Autodesk Fusion 360 part; units mm, degrees
(part 7 of 19)
  spline S237 degree 5 poles (-22.6635, 17.8166) (-22.6656, 17.8176) (-22.6751, 17.8223) (-22.6921, 17.8306) (-22.7166, 17.8424) (-22.7487, 17.8576) (-22.7863, 17.8752) (-22.824, 17.8925) (-22.8618, 17.9096) (-22.8998, 17.9265) (-22.938, 17.9432) (-22.9762, 17.9597) (-23.0146, 17.976) (-23.0531, 17.9922) (-23.0917, 18.0081) (-23.1305, 18.0238) (-23.1694, 18.0394) (-23.2084, 18.0547) (-23.2475, 18.0699) (-23.2867, 18.0849) (-23.3261, 18.0998) (-23.3655, 18.1144) (-23.405, 18.1289) (-23.4447, 18.1432) (-23.4845, 18.1574) (-23.5243, 18.1713) (-23.5643, 18.1851) (-23.6044, 18.1988) (-23.6445, 18.2123) (-23.6848, 18.2256) (-23.7251, 18.2388) (-23.7656, 18.2518) (-23.8061, 18.2646) (-23.8467, 18.2773) (-23.8874, 18.2899) (-23.9283, 18.3022) (-23.9692, 18.3145) (-24.0101, 18.3265) (-24.0512, 18.3385) (-24.0924, 18.3503) (-24.1336, 18.3619) (-24.1749, 18.3734) (-24.2163, 18.3847) (-24.2578, 18.3959) (-24.2994, 18.407) (-24.341, 18.4179) (-24.3827, 18.4286) (-24.4245, 18.4392) (-24.4664, 18.4497) (-24.5083, 18.46) (-24.5504, 18.4702) (-24.5925, 18.4803) (-24.6347, 18.4902) (-24.6769, 18.5) (-24.7192, 18.5096) (-24.7616, 18.5191) (-24.7956, 18.5266) (-24.8211, 18.5322) (-24.8381, 18.5358) (-24.8466, 18.5377) knots 0.224488 0.224488 0.224488 0.224488 0.224488 0.224488 0.228571 0.242857 0.257143 0.271429 0.285714 0.3 0.314286 0.328571 0.342857 0.357143 0.371429 0.385714 0.4 0.414286 0.428571 0.442857 0.457143 0.471429 0.485714 0.5 0.514286 0.528571 0.542857 0.557143 0.571429 0.585714 0.6 0.614286 0.628571 0.642857 0.657143 0.671429 0.685714 0.7 0.714286 0.728571 0.742857 0.757143 0.771429 0.785714 0.8 0.814286 0.828571 0.842857 0.857143 0.871429 0.885714 0.9 0.914286 0.928571 0.942857 0.957143 0.971429 0.985714 1 1 1 1 1 1
  arc A149 (-24.8466, 18.5377) -> (-25.3084, 17.9021) centre (0, 0) ccw
  spline S238 degree 5 poles (-25.3084, 17.9021) (-25.304, 17.8946) (-25.2953, 17.8795) (-25.2821, 17.857) (-25.2645, 17.827) (-25.2424, 17.7896) (-25.2201, 17.7523) (-25.1978, 17.7152) (-25.1753, 17.6781) (-25.1527, 17.6412) (-25.13, 17.6044) (-25.1072, 17.5677) (-25.0843, 17.5311) (-25.0613, 17.4946) (-25.0382, 17.4582) (-25.015, 17.422) (-24.9916, 17.3859) (-24.9682, 17.3499) (-24.9446, 17.314) (-24.9209, 17.2783) (-24.8971, 17.2426) (-24.8732, 17.2072) (-24.8491, 17.1718) (-24.825, 17.1365) (-24.8007, 17.1014) (-24.7763, 17.0664) (-24.7518, 17.0316) (-24.7272, 16.9969) (-24.7024, 16.9623) (-24.6776, 16.9278) (-24.6526, 16.8935) (-24.6275, 16.8594) (-24.6022, 16.8253) (-24.5769, 16.7915) (-24.5514, 16.7577) (-24.5258, 16.7241) (-24.5, 16.6907) (-24.4742, 16.6574) (-24.4482, 16.6242) (-24.422, 16.5913) (-24.3958, 16.5584) (-24.3694, 16.5258) (-24.3429, 16.4933) (-24.3162, 16.4609) (-24.2894, 16.4288) (-24.2625, 16.3967) (-24.2354, 16.3649) (-24.2081, 16.3333) (-24.1808, 16.3018) (-24.1532, 16.2705) (-24.1256, 16.2394) (-24.0977, 16.2085) (-24.0698, 16.1778) (-24.0416, 16.1473) (-24.0133, 16.117) (-23.9889, 16.0912) (-23.9701, 16.0715) (-23.957, 16.0579) (-23.9496, 16.0503) (-23.948, 16.0486) knots -1 -1 -1 -1 -1 -1 -0.985714 -0.971429 -0.957143 -0.942857 -0.928571 -0.914286 -0.9 -0.885714 -0.871429 -0.857143 -0.842857 -0.828571 -0.814286 -0.8 -0.785714 -0.771429 -0.757143 -0.742857 -0.728571 -0.714286 -0.7 -0.685714 -0.671429 -0.657143 -0.642857 -0.628571 -0.614286 -0.6 -0.585714 -0.571429 -0.557143 -0.542857 -0.528571 -0.514286 -0.5 -0.485714 -0.471429 -0.457143 -0.442857 -0.428571 -0.414286 -0.4 -0.385714 -0.371429 -0.357143 -0.342857 -0.328571 -0.314286 -0.3 -0.285714 -0.271429 -0.257143 -0.242857 -0.228571 -0.224488 -0.224488 -0.224488 -0.224488 -0.224488 -0.224488
  spline S239 degree 3 poles (-23.9365, 15.9236) (-23.9293, 15.9344) (-23.9242, 15.9466) (-23.9191, 15.9721) (-23.9191, 15.9853) (-23.9234, 16.0075) (-23.9266, 16.0167) (-23.9356, 16.0338) (-23.9412, 16.0417) (-23.948, 16.0486) knots 0 0 0 0 0.003906 0.003906 0.007813 0.007813 0.010709 0.010709 0.013605 0.013605 0.013605 0.013605
  arc A150 (-23.9365, 15.9236) -> (-24.2828, 15.3904) centre (0, 0) ccw
  spline S240 degree 3 poles (-24.4016, 15.35) (-24.3894, 15.3455) (-24.3764, 15.3435) (-24.3504, 15.3445) (-24.3376, 15.3475) (-24.317, 15.3569) (-24.3088, 15.3622) (-24.2943, 15.3748) (-24.2879, 15.3822) (-24.2828, 15.3904) knots 0 0 0 0 0.003906 0.003906 0.007813 0.007813 0.010709 0.010709 0.013605 0.013605 0.013605 0.013605
  spline S241 degree 5 poles (-24.4016, 15.35) (-24.4039, 15.3508) (-24.4138, 15.3545) (-24.4316, 15.3609) (-24.4572, 15.3701) (-24.4907, 15.3819) (-24.5299, 15.3954) (-24.5692, 15.4087) (-24.6087, 15.4218) (-24.6482, 15.4346) (-24.6879, 15.4473) (-24.7276, 15.4597) (-24.7675, 15.4719) (-24.8075, 15.4839) (-24.8476, 15.4957) (-24.8878, 15.5073) (-24.9281, 15.5187) (-24.9685, 15.5299) (-25.009, 15.5409) (-25.0495, 15.5517) (-25.0902, 15.5624) (-25.131, 15.5728) (-25.1718, 15.5831) (-25.2128, 15.5932) (-25.2538, 15.6031) (-25.2949, 15.6128) (-25.3361, 15.6224) (-25.3773, 15.6318) (-25.4187, 15.641) (-25.4601, 15.65) (-25.5016, 15.6589) (-25.5432, 15.6676) (-25.5849, 15.6762) (-25.6266, 15.6845) (-25.6684, 15.6927) (-25.7103, 15.7008) (-25.7522, 15.7087) (-25.7942, 15.7164) (-25.8363, 15.724) (-25.8785, 15.7314) (-25.9207, 15.7387) (-25.963, 15.7458) (-26.0054, 15.7527) (-26.0478, 15.7595) (-26.0903, 15.7661) (-26.1329, 15.7726) (-26.1755, 15.779) (-26.2181, 15.7852) (-26.2609, 15.7912) (-26.3037, 15.7971) (-26.3466, 15.8028) (-26.3895, 15.8084) (-26.4325, 15.8139) (-26.4755, 15.8192) (-26.5186, 15.8244) (-26.5617, 15.8294) (-26.5963, 15.8333) (-26.6223, 15.8361) (-26.6396, 15.838) (-26.6482, 15.8389) knots 0.224488 0.224488 0.224488 0.224488 0.224488 0.224488 0.228571 0.242857 0.257143 0.271429 0.285714 0.3 0.314286 0.328571 0.342857 0.357143 0.371429 0.385714 0.4 0.414286 0.428571 0.442857 0.457143 0.471429 0.485714 0.5 0.514286 0.528571 0.542857 0.557143 0.571429 0.585714 0.6 0.614286 0.628571 0.642857 0.657143 0.671429 0.685714 0.7 0.714286 0.728571 0.742857 0.757143 0.771429 0.785714 0.8 0.814286 0.828571 0.842857 0.857143 0.871429 0.885714 0.9 0.914286 0.928571 0.942857 0.957143 0.971429 0.985714 1 1 1 1 1 1
  arc A151 (-26.6482, 15.8389) -> (-27.041, 15.1586) centre (0, 0) ccw
  spline S242 degree 5 poles (-27.041, 15.1586) (-27.0359, 15.1515) (-27.0256, 15.1375) (-27.0102, 15.1164) (-26.9895, 15.0884) (-26.9636, 15.0536) (-26.9376, 15.0188) (-26.9115, 14.9842) (-26.8852, 14.9497) (-26.8589, 14.9154) (-26.8325, 14.8811) (-26.806, 14.847) (-26.7794, 14.813) (-26.7527, 14.7791) (-26.7259, 14.7454) (-26.699, 14.7118) (-26.672, 14.6783) (-26.6449, 14.645) (-26.6177, 14.6118) (-26.5904, 14.5787) (-26.563, 14.5457) (-26.5355, 14.5129) (-26.5079, 14.4803) (-26.4802, 14.4477) (-26.4524, 14.4154) (-26.4245, 14.3831) (-26.3965, 14.351) (-26.3684, 14.3191) (-26.3401, 14.2873) (-26.3118, 14.2556) (-26.2834, 14.2241) (-26.2548, 14.1927) (-26.2262, 14.1615) (-26.1974, 14.1305) (-26.1685, 14.0996) (-26.1396, 14.0689) (-26.1105, 14.0383) (-26.0813, 14.0079) (-26.0519, 13.9776) (-26.0225, 13.9476) (-25.993, 13.9177) (-25.9633, 13.8879) (-25.9335, 13.8584) (-25.9036, 13.829) (-25.8736, 13.7998) (-25.8435, 13.7708) (-25.8132, 13.742) (-25.7828, 13.7134) (-25.7523, 13.6849) (-25.7217, 13.6567) (-25.6909, 13.6287) (-25.66, 13.6008) (-25.6289, 13.5732) (-25.5978, 13.5458) (-25.5665, 13.5186) (-25.5395, 13.4955) (-25.5187, 13.4779) (-25.5043, 13.4658) (-25.4961, 13.459) (-25.4943, 13.4574) knots -1 -1 -1 -1 -1 -1 -0.985714 -0.971429 -0.957143 -0.942857 -0.928571 -0.914286 -0.9 -0.885714 -0.871429 -0.857143 -0.842857 -0.828571 -0.814286 -0.8 -0.785714 -0.771429 -0.757143 -0.742857 -0.728571 -0.714286 -0.7 -0.685714 -0.671429 -0.657143 -0.642857 -0.628571 -0.614286 -0.6 -0.585714 -0.571429 -0.557143 -0.542857 -0.528571 -0.514286 -0.5 -0.485714 -0.471429 -0.457143 -0.442857 -0.428571 -0.414286 -0.4 -0.385714 -0.371429 -0.357143 -0.342857 -0.328571 -0.314286 -0.3 -0.285714 -0.271429 -0.257143 -0.242857 -0.228571 -0.224488 -0.224488 -0.224488 -0.224488 -0.224488 -0.224488
  spline S243 degree 3 poles (-25.4698, 13.3343) (-25.4638, 13.3459) (-25.4601, 13.3585) (-25.4576, 13.3844) (-25.459, 13.3975) (-25.4656, 13.4192) (-25.4698, 13.4279) (-25.4804, 13.444) (-25.4869, 13.4513) (-25.4943, 13.4574) knots 0 0 0 0 0.003906 0.003906 0.007813 0.007813 0.010709 0.010709 0.013605 0.013605 0.013605 0.013605
  arc A152 (-25.4698, 13.3343) -> (-25.7585, 12.7678) centre (0, 0) ccw
  spline S244 degree 3 poles (-25.8725, 12.7152) (-25.8598, 12.7121) (-25.8467, 12.7114) (-25.8209, 12.7151) (-25.8085, 12.7194) (-25.789, 12.731) (-25.7814, 12.737) (-25.7683, 12.7512) (-25.7628, 12.7592) (-25.7585, 12.7678) knots 0 0 0 0 0.003906 0.003906 0.007813 0.007813 0.010709 0.010709 0.013605 0.013605 0.013605 0.013605
  spline S245 degree 5 poles (-25.8725, 12.7152) (-25.8748, 12.7158) (-25.8851, 12.7184) (-25.9034, 12.723) (-25.9299, 12.7294) (-25.9644, 12.7377) (-26.0048, 12.747) (-26.0453, 12.7561) (-26.0859, 12.765) (-26.1265, 12.7736) (-26.1673, 12.7821) (-26.2082, 12.7902) (-26.2491, 12.7982) (-26.2901, 12.806) (-26.3312, 12.8135) (-26.3724, 12.8209) (-26.4137, 12.828) (-26.455, 12.8349) (-26.4964, 12.8416) (-26.5379, 12.8482) (-26.5795, 12.8545) (-26.6211, 12.8606) (-26.6628, 12.8666) (-26.7046, 12.8723) (-26.7464, 12.8779) (-26.7883, 12.8833) (-26.8303, 12.8885) (-26.8723, 12.8935) (-26.9144, 12.8983) (-26.9565, 12.903) (-26.9987, 12.9075) (-27.041, 12.9118) (-27.0833, 12.9159) (-27.1257, 12.9199) (-27.1681, 12.9237) (-27.2106, 12.9273) (-27.2532, 12.9308) (-27.2958, 12.9341) (-27.3384, 12.9372) (-27.3811, 12.9402) (-27.4239, 12.943) (-27.4667, 12.9456) (-27.5095, 12.9481) (-27.5524, 12.9504) (-27.5954, 12.9526) (-27.6384, 12.9546) (-27.6814, 12.9565) (-27.7245, 12.9581) (-27.7677, 12.9597) (-27.8108, 12.9611) (-27.8541, 12.9623) (-27.8973, 12.9634) (-27.9407, 12.9643) (-27.984, 12.9651) (-28.0274, 12.9657) (-28.0708, 12.9662) (-28.1056, 12.9665) (-28.1317, 12.9666) (-28.1492, 12.9667) (-28.1579, 12.9667) knots 0.224488 0.224488 0.224488 0.224488 0.224488 0.224488 0.228571 0.242857 0.257143 0.271429 0.285714 0.3 0.314286 0.328571 0.342857 0.357143 0.371429 0.385714 0.4 0.414286 0.428571 0.442857 0.457143 0.471429 0.485714 0.5 0.514286 0.528571 0.542857 0.557143 0.571429 0.585714 0.6 0.614286 0.628571 0.642857 0.657143 0.671429 0.685714 0.7 0.714286 0.728571 0.742857 0.757143 0.771429 0.785714 0.8 0.814286 0.828571 0.842857 0.857143 0.871429 0.885714 0.9 0.914286 0.928571 0.942857 0.957143 0.971429 0.985714 1 1 1 1 1 1
  arc A153 (-28.1579, 12.9667) -> (-28.4774, 12.249) centre (0, 0) ccw
  spline S246 degree 5 poles (-28.4774, 12.249) (-28.4716, 12.2425) (-28.4599, 12.2296) (-28.4423, 12.2103) (-28.4188, 12.1846) (-28.3894, 12.1527) (-28.3599, 12.1208) (-28.3303, 12.0891) (-28.3006, 12.0576) (-28.2709, 12.0261) (-28.241, 11.9948) (-28.2111, 11.9637) (-28.1811, 11.9326) (-28.151, 11.9018) (-28.1208, 11.871) (-28.0906, 11.8404) (-28.0602, 11.8099) (-28.0298, 11.7796) (-27.9993, 11.7494) (-27.9687, 11.7194) (-27.938, 11.6895) (-27.9072, 11.6597) (-27.8763, 11.6301) (-27.8454, 11.6007) (-27.8143, 11.5714) (-27.7832, 11.5422) (-27.752, 11.5132) (-27.7207, 11.4844) (-27.6893, 11.4557) (-27.6578, 11.4272) (-27.6262, 11.3988) (-27.5946, 11.3706) (-27.5628, 11.3426) (-27.5309, 11.3147) (-27.499, 11.287) (-27.467, 11.2595) (-27.4348, 11.2321) (-27.4026, 11.2049) (-27.3703, 11.1779) (-27.3379, 11.1511) (-27.3054, 11.1244) (-27.2728, 11.098) (-27.2401, 11.0717) (-27.2073, 11.0456) (-27.1743, 11.0197) (-27.1413, 10.994) (-27.1082, 10.9685) (-27.075, 10.9432) (-27.0417, 10.9181) (-27.0083, 10.8932) (-26.9747, 10.8686) (-26.9411, 10.8441) (-26.9073, 10.8199) (-26.8735, 10.7959) (-26.8395, 10.7721) (-26.8103, 10.752) (-26.7878, 10.7367) (-26.7721, 10.7261) (-26.7633, 10.7202) (-26.7613, 10.7188) knots -1 -1 -1 -1 -1 -1 -0.985714 -0.971429 -0.957143 -0.942857 -0.928571 -0.914286 -0.9 -0.885714 -0.871429 -0.857143 -0.842857 -0.828571 -0.814286 -0.8 -0.785714 -0.771429 -0.757143 -0.742857 -0.728571 -0.714286 -0.7 -0.685714 -0.671429 -0.657143 -0.642857 -0.628571 -0.614286 -0.6 -0.585714 -0.571429 -0.557143 -0.542857 -0.528571 -0.514286 -0.5 -0.485714 -0.471429 -0.457143 -0.442857 -0.428571 -0.414286 -0.4 -0.385714 -0.371429 -0.357143 -0.342857 -0.328571 -0.314286 -0.3 -0.285714 -0.271429 -0.257143 -0.242857 -0.228571 -0.224488 -0.224488 -0.224488 -0.224488 -0.224488 -0.224488
  spline S247 degree 3 poles (-26.7241, 10.599) (-26.7193, 10.6111) (-26.7169, 10.624) (-26.7172, 10.65) (-26.7199, 10.6629) (-26.7288, 10.6838) (-26.7338, 10.6921) (-26.7461, 10.7069) (-26.7533, 10.7135) (-26.7613, 10.7188) knots 0 0 0 0 0.003906 0.003906 0.007813 0.007813 0.010709 0.010709 0.013605 0.013605 0.013605 0.013605
  arc A154 (-26.7241, 10.599) -> (-26.952, 10.0054) centre (0, 0) ccw
  spline S248 degree 3 poles (-27.0598, 9.9412) (-27.047, 9.9393) (-27.0338, 9.94) (-27.0086, 9.9464) (-26.9967, 9.952) (-26.9785, 9.9655) (-26.9716, 9.9724) (-26.96, 9.9878) (-26.9553, 9.9963) (-26.952, 10.0054) knots 0 0 0 0 0.003906 0.003906 0.007813 0.007813 0.010709 0.010709 0.013605 0.013605 0.013605 0.013605
  spline S249 degree 5 poles (-27.0598, 9.9412) (-27.0622, 9.9415) (-27.0727, 9.943) (-27.0914, 9.9456) (-27.1184, 9.9493) (-27.1536, 9.9539) (-27.1948, 9.9589) (-27.236, 9.9638) (-27.2773, 9.9683) (-27.3186, 9.9727) (-27.3601, 9.9768) (-27.4015, 9.9807) (-27.4431, 9.9843) (-27.4847, 9.9878) (-27.5264, 9.991) (-27.5681, 9.994) (-27.6099, 9.9967) (-27.6517, 9.9993) (-27.6936, 10.0016) (-27.7355, 10.0038) (-27.7775, 10.0057) (-27.8196, 10.0075) (-27.8617, 10.0091) (-27.9038, 10.0104) (-27.946, 10.0116) (-27.9882, 10.0126) (-28.0305, 10.0133) (-28.0728, 10.0139) (-28.1152, 10.0144) (-28.1576, 10.0146) (-28.2, 10.0146) (-28.2425, 10.0145) (-28.285, 10.0142) (-28.3276, 10.0137) (-28.3702, 10.0131) (-28.4128, 10.0122) (-28.4555, 10.0112) (-28.4982, 10.01) (-28.541, 10.0087) (-28.5837, 10.0072) (-28.6265, 10.0055) (-28.6694, 10.0037) (-28.7123, 10.0016) (-28.7552, 9.9995) (-28.7981, 9.9971) (-28.8411, 9.9946) (-28.8841, 9.992) (-28.9271, 9.9892) (-28.9702, 9.9862) (-29.0133, 9.983) (-29.0564, 9.9798) (-29.0996, 9.9763) (-29.1427, 9.9727) (-29.1859, 9.9689) (-29.2292, 9.965) (-29.2724, 9.961) (-29.307, 9.9576) (-29.333, 9.955) (-29.3503, 9.9532) (-29.359, 9.9524) knots 0.224488 0.224488 0.224488 0.224488 0.224488 0.224488 0.228571 0.242857 0.257143 0.271429 0.285714 0.3 0.314286 0.328571 0.342857 0.357143 0.371429 0.385714 0.4 0.414286 0.428571 0.442857 0.457143 0.471429 0.485714 0.5 0.514286 0.528571 0.542857 0.557143 0.571429 0.585714 0.6 0.614286 0.628571 0.642857 0.657143 0.671429 0.685714 0.7 0.714286 0.728571 0.742857 0.757143 0.771429 0.785714 0.8 0.814286 0.828571 0.842857 0.857143 0.871429 0.885714 0.9 0.914286 0.928571 0.942857 0.957143 0.971429 0.985714 1 1 1 1 1 1
  arc A155 (-29.359, 9.9524) -> (-29.6018, 9.2052) centre (0, 0) ccw
  spline S250 degree 5 poles (-29.6018, 9.2052) (-29.5953, 9.1994) (-29.5823, 9.1877) (-29.5628, 9.1704) (-29.5368, 9.1473) (-29.5042, 9.1186) (-29.4715, 9.09) (-29.4388, 9.0616) (-29.406, 9.0333) (-29.3731, 9.0051) (-29.3401, 8.9771) (-29.3071, 8.9493) (-29.274, 8.9215) (-29.2409, 8.894) (-29.2076, 8.8665) (-29.1743, 8.8393) (-29.141, 8.8121) (-29.1075, 8.7851) (-29.074, 8.7583) (-29.0405, 8.7316) (-29.0068, 8.7051) (-28.9731, 8.6787) (-28.9393, 8.6525) (-28.9054, 8.6265) (-28.8715, 8.6006) (-28.8375, 8.5748) (-28.8034, 8.5493) (-28.7693, 8.5239) (-28.735, 8.4986) (-28.7007, 8.4735) (-28.6664, 8.4486) (-28.6319, 8.4239) (-28.5974, 8.3993) (-28.5628, 8.3749) (-28.5282, 8.3507) (-28.4934, 8.3267) (-28.4586, 8.3028) (-28.4237, 8.2792) (-28.3888, 8.2557) (-28.3537, 8.2324) (-28.3186, 8.2093) (-28.2834, 8.1864) (-28.2481, 8.1637) (-28.2128, 8.1412) (-28.1774, 8.1188) (-28.1418, 8.0967) (-28.1062, 8.0748) (-28.0706, 8.0531) (-28.0348, 8.0317) (-27.999, 8.0104) (-27.963, 7.9894) (-27.927, 7.9686) (-27.8909, 7.9481) (-27.8547, 7.9277) (-27.8185, 7.9076) (-27.7873, 7.8907) (-27.7633, 7.8778) (-27.7466, 7.8689) (-27.7372, 7.8639) (-27.7352, 7.8628) knots -1 -1 -1 -1 -1 -1 -0.985714 -0.971429 -0.957143 -0.942857 -0.928571 -0.914286 -0.9 -0.885714 -0.871429 -0.857143 -0.842857 -0.828571 -0.814286 -0.8 -0.785714 -0.771429 -0.757143 -0.742857 -0.728571 -0.714286 -0.7 -0.685714 -0.671429 -0.657143 -0.642857 -0.628571 -0.614286 -0.6 -0.585714 -0.571429 -0.557143 -0.542857 -0.528571 -0.514286 -0.5 -0.485714 -0.471429 -0.457143 -0.442857 -0.428571 -0.414286 -0.4 -0.385714 -0.371429 -0.357143 -0.342857 -0.328571 -0.314286 -0.3 -0.285714 -0.271429 -0.257143 -0.242857 -0.228571 -0.224488 -0.224488 -0.224488 -0.224488 -0.224488 -0.224488
  spline S251 degree 3 poles (-27.6856, 7.7475) (-27.6821, 7.76) (-27.6811, 7.7731) (-27.6841, 7.799) (-27.6881, 7.8115) (-27.6991, 7.8313) (-27.705, 7.839) (-27.7188, 7.8526) (-27.7266, 7.8583) (-27.7352, 7.8628) knots 0 0 0 0 0.003906 0.003906 0.007813 0.007813 0.010709 0.010709 0.013605 0.013605 0.013605 0.013605
  arc A156 (-27.6856, 7.7475) -> (-27.8502, 7.1333) centre (0, 0) ccw
  spline S252 degree 3 poles (-27.9507, 7.0582) (-27.9377, 7.0577) (-27.9248, 7.0598) (-27.9003, 7.0688) (-27.8891, 7.0756) (-27.8724, 7.0909) (-27.8662, 7.0984) (-27.8563, 7.115) (-27.8526, 7.124) (-27.8502, 7.1333) knots 0 0 0 0 0.003906 0.003906 0.007813 0.007813 0.010709 0.010709 0.013605 0.013605 0.013605 0.013605
  spline S253 degree 5 poles (-27.9507, 7.0582) (-27.9531, 7.0583) (-27.9637, 7.0587) (-27.9826, 7.0593) (-28.0098, 7.0601) (-28.0453, 7.061) (-28.0868, 7.0618) (-28.1283, 7.0622) (-28.1698, 7.0625) (-28.2114, 7.0625) (-28.253, 7.0622) (-28.2947, 7.0618) (-28.3364, 7.0611) (-28.3781, 7.0601) (-28.4199, 7.059) (-28.4617, 7.0576) (-28.5036, 7.0559) (-28.5454, 7.0541) (-28.5873, 7.0521) (-28.6293, 7.0498) (-28.6712, 7.0474) (-28.7132, 7.0447) (-28.7553, 7.0419) (-28.7973, 7.0388) (-28.8394, 7.0356) (-28.8815, 7.0321) (-28.9236, 7.0285) (-28.9658, 7.0247) (-29.0079, 7.0207) (-29.0501, 7.0165) (-29.0923, 7.0121) (-29.1346, 7.0075) (-29.1768, 7.0027) (-29.2191, 6.9978) (-29.2614, 6.9927) (-29.3037, 6.9874) (-29.3461, 6.982) (-29.3884, 6.9763) (-29.4308, 6.9705) (-29.4732, 6.9646) (-29.5156, 6.9584) (-29.558, 6.9521) (-29.6004, 6.9456) (-29.6429, 6.939) (-29.6854, 6.9321) (-29.7278, 6.9252) (-29.7703, 6.918) (-29.8128, 6.9107) (-29.8553, 6.9033) (-29.8979, 6.8956) (-29.9404, 6.8879) (-29.983, 6.8799) (-30.0255, 6.8718) (-30.0681, 6.8636) (-30.1107, 6.8552) (-30.1533, 6.8466) (-30.1873, 6.8396) (-30.2129, 6.8343) (-30.2299, 6.8308) (-30.2385, 6.829) knots 0.224488 0.224488 0.224488 0.224488 0.224488 0.224488 0.228571 0.242857 0.257143 0.271429 0.285714 0.3 0.314286 0.328571 0.342857 0.357143 0.371429 0.385714 0.4 0.414286 0.428571 0.442857 0.457143 0.471429 0.485714 0.5 0.514286 0.528571 0.542857 0.557143 0.571429 0.585714 0.6 0.614286 0.628571 0.642857 0.657143 0.671429 0.685714 0.7 0.714286 0.728571 0.742857 0.757143 0.771429 0.785714 0.8 0.814286 0.828571 0.842857 0.857143 0.871429 0.885714 0.9 0.914286 0.928571 0.942857 0.957143 0.971429 0.985714 1 1 1 1 1 1
  arc A157 (-30.2385, 6.829) -> (-30.4018, 6.0605) centre (0, 0) ccw
  spline S254 degree 5 poles (-30.4018, 6.0605) (-30.3948, 6.0554) (-30.3806, 6.0452) (-30.3594, 6.03) (-30.3311, 6.0097) (-30.2957, 5.9846) (-30.2602, 5.9596) (-30.2247, 5.9348) (-30.1891, 5.91) (-30.1535, 5.8855) (-30.1178, 5.8611) (-30.082, 5.8368) (-30.0462, 5.8127) (-30.0104, 5.7887) (-29.9744, 5.7649) (-29.9385, 5.7413) (-29.9025, 5.7178) (-29.8664, 5.6945) (-29.8303, 5.6713) (-29.7941, 5.6483) (-29.7578, 5.6254) (-29.7215, 5.6027) (-29.6852, 5.5802) (-29.6488, 5.5578) (-29.6123, 5.5356) (-29.5758, 5.5135) (-29.5393, 5.4917) (-29.5026, 5.47) (-29.466, 5.4484) (-29.4292, 5.4271) (-29.3925, 5.4059) (-29.3556, 5.3849) (-29.3187, 5.3641) (-29.2818, 5.3434) (-29.2448, 5.323) (-29.2077, 5.3027) (-29.1706, 5.2826) (-29.1334, 5.2627) (-29.0962, 5.243) (-29.0589, 5.2235) (-29.0216, 5.2042) (-28.9842, 5.1851) (-28.9467, 5.1662) (-28.9092, 5.1475) (-28.8716, 5.129) (-28.834, 5.1107) (-28.7963, 5.0927) (-28.7586, 5.0749) (-28.7208, 5.0572) (-28.6829, 5.0399) (-28.645, 5.0227) (-28.607, 5.0058) (-28.5689, 4.9891) (-28.5308, 4.9727) (-28.4926, 4.9565) (-28.4599, 4.9429) (-28.4347, 4.9326) (-28.4172, 4.9255) (-28.4073, 4.9215) (-28.4051, 4.9206) knots -1 -1 -1 -1 -1 -1 -0.985714 -0.971429 -0.957143 -0.942857 -0.928571 -0.914286 -0.9 -0.885714 -0.871429 -0.857143 -0.842857 -0.828571 -0.814286 -0.8 -0.785714 -0.771429 -0.757143 -0.742857 -0.728571 -0.714286 -0.7 -0.685714 -0.671429 -0.657143 -0.642857 -0.628571 -0.614286 -0.6 -0.585714 -0.571429 -0.557143 -0.542857 -0.528571 -0.514286 -0.5 -0.485714 -0.471429 -0.457143 -0.442857 -0.428571 -0.414286 -0.4 -0.385714 -0.371429 -0.357143 -0.342857 -0.328571 -0.314286 -0.3 -0.285714 -0.271429 -0.257143 -0.242857 -0.228571 -0.224488 -0.224488 -0.224488 -0.224488 -0.224488 -0.224488
  spline S255 degree 3 poles (-28.3438, 4.8111) (-28.3416, 4.8239) (-28.342, 4.8371) (-28.3477, 4.8625) (-28.353, 4.8745) (-28.366, 4.8931) (-28.3726, 4.9001) (-28.3878, 4.9121) (-28.3961, 4.917) (-28.4051, 4.9206) knots 0 0 0 0 0.003906 0.003906 0.007813 0.007813 0.010709 0.010709 0.013605 0.013605 0.013605 0.013605
  arc A158 (-28.3438, 4.8111) -> (-28.4432, 4.1831) centre (0, 0) ccw
  spline S256 degree 3 poles (-28.5354, 4.0979) (-28.5224, 4.0988) (-28.5097, 4.1022) (-28.4864, 4.1137) (-28.4759, 4.1216) (-28.4609, 4.1386) (-28.4556, 4.1467) (-28.4474, 4.1642) (-28.4447, 4.1735) (-28.4432, 4.1831) knots 0 0 0 0 0.003906 0.003906 0.007813 0.007813 0.010709 0.010709 0.013605 0.013605 0.013605 0.013605
  spline S257 degree 5 poles (-28.5354, 4.0979) (-28.5378, 4.0977) (-28.5484, 4.097) (-28.5672, 4.0957) (-28.5944, 4.0936) (-28.6298, 4.0908) (-28.6711, 4.0872) (-28.7124, 4.0833) (-28.7537, 4.0792) (-28.7951, 4.0749) (-28.8365, 4.0703) (-28.8778, 4.0655) (-28.9192, 4.0604) (-28.9607, 4.0551) (-29.0021, 4.0496) (-29.0435, 4.0438) (-29.085, 4.0379) (-29.1264, 4.0317) (-29.1679, 4.0253) (-29.2094, 4.0186) (-29.2508, 4.0118) (-29.2923, 4.0048) (-29.3338, 3.9976) (-29.3753, 3.9901) (-29.4168, 3.9825) (-29.4583, 3.9747) (-29.4998, 3.9667) (-29.5414, 3.9584) (-29.5829, 3.95) (-29.6244, 3.9415) (-29.6659, 3.9327) (-29.7075, 3.9237) (-29.749, 3.9146) (-29.7905, 3.9053) (-29.8321, 3.8958) (-29.8736, 3.8861) (-29.9151, 3.8762) (-29.9567, 3.8662) (-29.9982, 3.856) (-30.0397, 3.8456) (-30.0812, 3.8351) (-30.1228, 3.8244) (-30.1643, 3.8135) (-30.2058, 3.8024) (-30.2473, 3.7912) (-30.2889, 3.7798) (-30.3304, 3.7683) (-30.3719, 3.7566) (-30.4134, 3.7447) (-30.4549, 3.7327) (-30.4964, 3.7205) (-30.5379, 3.7082) (-30.5793, 3.6957) (-30.6208, 3.683) (-30.6623, 3.6702) (-30.7037, 3.6572) (-30.7369, 3.6467) (-30.7618, 3.6388) (-30.7784, 3.6335) (-30.7866, 3.6308) knots 0.224488 0.224488 0.224488 0.224488 0.224488 0.224488 0.228571 0.242857 0.257143 0.271429 0.285714 0.3 0.314286 0.328571 0.342857 0.357143 0.371429 0.385714 0.4 0.414286 0.428571 0.442857 0.457143 0.471429 0.485714 0.5 0.514286 0.528571 0.542857 0.557143 0.571429 0.585714 0.6 0.614286 0.628571 0.642857 0.657143 0.671429 0.685714 0.7 0.714286 0.728571 0.742857 0.757143 0.771429 0.785714 0.8 0.814286 0.828571 0.842857 0.857143 0.871429 0.885714 0.9 0.914286 0.928571 0.942857 0.957143 0.971429 0.985714 1 1 1 1 1 1
  arc A159 (-30.7866, 3.6308) -> (-30.8688, 2.8495) centre (0, 0) ccw
  spline S258 degree 5 poles (-30.8688, 2.8495) (-30.8612, 2.8451) (-30.8461, 2.8365) (-30.8234, 2.8235) (-30.7932, 2.8064) (-30.7553, 2.7851) (-30.7174, 2.7639) (-30.6795, 2.7429) (-30.6415, 2.722) (-30.6035, 2.7013) (-30.5654, 2.6808) (-30.5273, 2.6604) (-30.4892, 2.6402) (-30.451, 2.6201) (-30.4128, 2.6002) (-30.3746, 2.5804) (-30.3363, 2.5608) (-30.298, 2.5414) (-30.2596, 2.5221) (-30.2213, 2.503) (-30.1828, 2.484) (-30.1444, 2.4653) (-30.1059, 2.4466) (-30.0673, 2.4282) (-30.0287, 2.4099) (-29.9901, 2.3918) (-29.9515, 2.3739) (-29.9128, 2.3561) (-29.8741, 2.3386) (-29.8353, 2.3212) (-29.7965, 2.3039) (-29.7577, 2.2869) (-29.7188, 2.2701) (-29.6799, 2.2534) (-29.641, 2.2369) (-29.602, 2.2206) (-29.563, 2.2045) (-29.5239, 2.1886) (-29.4849, 2.1729) (-29.4457, 2.1574) (-29.4066, 2.1421) (-29.3674, 2.127) (-29.3282, 2.1122) (-29.2889, 2.0975) (-29.2496, 2.083) (-29.2103, 2.0688) (-29.1709, 2.0548) (-29.1315, 2.041) (-29.0921, 2.0274) (-29.0526, 2.0141) (-29.0131, 2.001) (-28.9735, 1.9881) (-28.9339, 1.9755) (-28.8943, 1.9632) (-28.8546, 1.9511) (-28.8206, 1.9409) (-28.7945, 1.9333) (-28.7763, 1.9281) (-28.7661, 1.9252) (-28.7638, 1.9245) knots -1 -1 -1 -1 -1 -1 -0.985714 -0.971429 -0.957143 -0.942857 -0.928571 -0.914286 -0.9 -0.885714 -0.871429 -0.857143 -0.842857 -0.828571 -0.814286 -0.8 -0.785714 -0.771429 -0.757143 -0.742857 -0.728571 -0.714286 -0.7 -0.685714 -0.671429 -0.657143 -0.642857 -0.628571 -0.614286 -0.6 -0.585714 -0.571429 -0.557143 -0.542857 -0.528571 -0.514286 -0.5 -0.485714 -0.471429 -0.457143 -0.442857 -0.428571 -0.414286 -0.4 -0.385714 -0.371429 -0.357143 -0.342857 -0.328571 -0.314286 -0.3 -0.285714 -0.271429 -0.257143 -0.242857 -0.228571 -0.224488 -0.224488 -0.224488 -0.224488 -0.224488 -0.224488
  spline S259 degree 3 poles (-28.6914, 1.822) (-28.6906, 1.835) (-28.6923, 1.848) (-28.7006, 1.8727) (-28.7072, 1.8841) (-28.7221, 1.9012) (-28.7294, 1.9075) (-28.7457, 1.9179) (-28.7546, 1.9219) (-28.7638, 1.9245) knots 0 0 0 0 0.003906 0.003906 0.007813 0.007813 0.010709 0.010709 0.013605 0.013605 0.013605 0.013605
  line L20 (0, 31) -> (0, 3.7492)
  line L21 (2.2037, 3.0332) -> (18.2213, 25.0795)
  circle A160 centre (0, 0) radius 7.5
  circle A161 centre (0, 0) radius 27.5
  dimension "d19" = 36
  dimension "d20" = 15
  dimension "d21" = 55
  constraint vertical L20
  constraint coincident A1.centre L20
  constraint coincident A1.centre L21
  constraint coincident A9 L20.end
  constraint coincident A13 L21.start
  constraint coincident A131 L20.start
  constraint coincident A119 L21.end
  constraint coincident A1.centre A3.centre
  constraint concentric A1 A161
  measures "d19" angle of L20 L21
  measures "d20" diameter of A160
  measures "d21" diameter of A161
extrude "Estrusione4" cut sketch "Schizzo1 (3)" against normal blind 1 contours L20 L21 A160 A161 picked at (8.9949, 18.7465) bodies 1 in component "Spur Gear (60 teeth)"
pattern_circular "Serie C2" count 5 over 360 about axis through (0, 0, 0) along (0, 0, 1) of "Estrusione4" in component "Spur Gear (60 teeth)"
extrude "Estrusione5" cut 1 faces at (-3.6482, -2.3787, 8) along direction (0, 0, -1) blind 1.6 on bodies 1 bodies 1 in component "Spur Gear (60 teeth)"
sketch "Schizzo2 (3)" plane through (0, 0, 2) normal (0, 0, 1) x (-1, 0, 0)
  line L0 (7.1329, -2.3176) -> (26.1541, -8.498)
  arc A0 (26.1541, -8.498) -> (26.1541, 8.498) centre (0, 0) ccw
  line L1 (26.1541, 8.498) -> (7.1329, 2.3176)
  arc A1 (7.1329, -2.3176) -> (7.1329, 2.3176) centre (0, 0) ccw
  line L2 (24.4009, 8.0452) -> (-1.5991, 8.0452) construction
  line L3 (-1.5991, 8.0452) -> (-1.5991, -2.9548) construction
  line L4 (-1.5991, -2.9548) -> (24.4009, -2.9548) construction
  line L5 (24.4009, -2.9548) -> (24.4009, 8.0452) construction
  dimension "d28" = 5
  text T0 "60s" font "Arial" height 5 bold align left top in box 26 x 11 at (24.4009, 8.0452) x (-1, 0) y (0, -1) spacing 1 kerned
extrude "Estrusione6" add sketch "Schizzo2 (3)" along normal blind 1 text T0 bodies 1 in component "Spur Gear (60 teeth)"
component "Spur Gear (60 teeth)" placed x (1, 0, 0) y (0, 1, 0) z (0, 0, 1) at (0, 0, 0)
component "Spur Gear (10 teeth)" placed x (1, 0, 0) y (0, 1, 0) z (0, 0, 1) at (0, 0, 0)
equation "d19 = ( 360 / 10 ) * 1 deg"

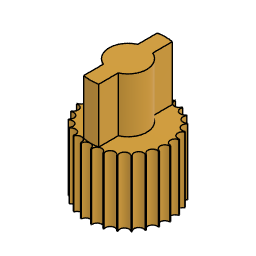
design "2 pomello lancetta secondi"
Autodesk Fusion 360 part; units mm, degrees
sketch "Schizzo1" plane through (0, 0, 0) normal (0, 0, 1) x (1, 0, 0)
  line L0 (0, -45) -> (5, 0)
  line L1 (5, 0) -> (0, 15)
  line L2 (0, 15) -> (-5, 0)
  line L3 (-5, 0) -> (0, -45)
  line L4 (0, -45) -> (0, 15) construction
  line L5 (5, 0) -> (-5, 0) construction
  line L6 (-1, 15) -> (1, 15)
  line L7 (1, 15) -> (1, -45)
  line L8 (1, -45) -> (-1, -45)
  line L9 (-1, -45) -> (-1, 15)
  circle A0 centre (0, 0) radius 5
  dimension "d1" = 45
  dimension "d2" = 15
  dimension "d3" = 5
  dimension "d12" = 1
  dimension "d13" = 1
  constraint vertical L4
  constraint perpendicular L4 L5
  constraint midpoint A0.centre L5
  constraint equal L0 L3
  constraint equal L1 L2
  constraint horizontal L6
  constraint vertical L7
  constraint horizontal L8
  constraint vertical L9
  constraint coincident A0.centre origin
  constraint coincident L0.end A0
  constraint midpoint L0.start L8
  constraint midpoint L1.end L6
  measures "d1" vertical distance of L0.start L0.end
  measures "d2" vertical distance of L0.end L1.end
  measures "d3" horizontal distance of L0.start L0.end
  measures "d12" distance of A0.centre L9
  measures "d13" distance of A0.centre L7
extrude "Estrusione1" add sketch "Schizzo1" along normal blind 2 contours L0 L3 L7 L9 A0 | L3 L8 L9 | L0 L7 L8 | L0 L1 L7 A0 | L0 A0 | L7 L9 A0 | L3 A0 | L2 L3 L9 A0 | L1 A0 | L1 L2 L7 L9 A0 | L2 A0 | L1 L6 L7 | L2 L6 L9
sketch "Schizzo2" plane through (0, 0, 2) normal (0, 0, 1) x (-1, 0, 0)
  circle A0 centre (0, 0) radius 2
  circle A1 centre (0, 0) radius 4
  line L0 (-0.8, 24) -> (0.8, 24)
  line L1 (0.8, 24) -> (0.8, -21)
  line L2 (0.8, -21) -> (-0.8, -21)
  line L3 (-0.8, -21) -> (-0.8, 24)
  arc A2 (-1, 4.899) -> (-1, -4.899) centre (0, 0) ccw
  line L4 (-1, -4.899) -> (-1, -15)
  line L5 (-1, -15) -> (1, -15)
  line L6 (1, -15) -> (1, -4.899)
  arc A3 (1, -4.899) -> (1, 4.899) centre (0, 0) ccw
  line L7 (1, 4.899) -> (1, 45)
  line L8 (-1, 45) -> (-1, 4.899)
  line L9 (1, 45) -> (-1, 45)
  dimension "d6" = 4
  dimension "d7" = 8
  dimension "d8" = 0.8
  dimension "d9" = 0.8
  constraint coincident A0.centre A1.centre
  constraint horizontal L0
  constraint vertical L1
  constraint horizontal L2
  constraint vertical L3
  measures "d6" diameter of A0
  measures "d7" diameter of A1
  measures "d8" distance of A0.centre L3
  measures "d9" distance of A0.centre L1
extrude "Estrusione2" add sketch "Schizzo2" along normal blind 3.8 contours A0 L1 | A0 L1 L3 | A0 A1 L1 L3 | A0 A1 L1 L3 | A0 L3
extrude "Estrusione3" add 1 faces at (0.3333, -45, 0.6667) along direction (0, -1, 0) blind 10
sketch "Schizzo3" plane through (0, 0, 0) normal (0, 0, -1) x (1, 0, 0)
  line L0 (1, 4.899) -> (1, 55)
  line L1 (1, 55) -> (-1, 55)
  line L2 (-1, 55) -> (-1, 4.899)
  arc A0 (-1, 4.899) -> (-1, -4.899) centre (0, 0) ccw
  line L3 (-1, -4.899) -> (-1, -15)
  line L4 (-1, -15) -> (1, -15)
  line L5 (1, -15) -> (1, -4.899)
  arc A1 (1, -4.899) -> (1, 4.899) centre (0, 0) ccw
  circle A2 centre (0, 0) radius 6
  dimension "d16" = 12
  constraint concentric A0 A2
  measures "d16" diameter of A2
extrude "Estrusione4" add sketch "Schizzo3" against normal up to surface (2 mm away) contours L0 L5 A1 A2 | L2 A0 L3 A2
sketch "Schizzo4" plane through (0, 0, 0) normal (0, 0, -1) x (1, 0, 0)
  line L0 (1, 5.9161) -> (1, 55)
  line L1 (1, 55) -> (-1, 55)
  line L2 (-1, 55) -> (-1, 5.9161)
  arc A0 (-1, 5.9161) -> (-1, -5.9161) centre (0, 0) ccw
  line L3 (-1, -5.9161) -> (-1, -15)
  line L4 (-1, -15) -> (1, -15)
  line L5 (1, -15) -> (1, -5.9161)
  arc A1 (1, -5.9161) -> (1, 5.9161) centre (0, 0) ccw
  circle A2 centre (0, 0) radius 4.5
  circle A3 centre (0, 4.5) radius 0.5
  circle A4 centre (-1.0769, 4.3692) radius 0.5
  circle A5 centre (-2.0913, 3.9846) radius 0.5
  circle A6 centre (-2.9841, 3.3683) radius 0.5
  circle A7 centre (-3.7034, 2.5563) radius 0.5
  circle A8 centre (-4.2076, 1.5957) radius 0.5
  circle A9 centre (-4.4672, 0.5424) radius 0.5
  circle A10 centre (-4.4672, -0.5424) radius 0.5
  circle A11 centre (-4.2076, -1.5957) radius 0.5
  circle A12 centre (-3.7034, -2.5563) radius 0.5
  circle A13 centre (-2.9841, -3.3683) radius 0.5
  circle A14 centre (-2.0913, -3.9846) radius 0.5
  circle A15 centre (-1.0769, -4.3692) radius 0.5
  circle A16 centre (0, -4.5) radius 0.5
  circle A17 centre (1.0769, -4.3692) radius 0.5
  circle A18 centre (2.0913, -3.9846) radius 0.5
  circle A19 centre (2.9841, -3.3683) radius 0.5
  circle A20 centre (3.7034, -2.5563) radius 0.5
  circle A21 centre (4.2076, -1.5957) radius 0.5
  circle A22 centre (4.4672, -0.5424) radius 0.5
  circle A23 centre (4.4672, 0.5424) radius 0.5
  circle A24 centre (4.2076, 1.5957) radius 0.5
  circle A25 centre (3.7034, 2.5563) radius 0.5
  circle A26 centre (2.9841, 3.3683) radius 0.5
  circle A27 centre (2.0913, 3.9846) radius 0.5
  circle A28 centre (1.0769, 4.3692) radius 0.5
  dimension "d19" = 9
  dimension "d20" = 1
  dimension "d22" = 360
  constraint coincident A0.centre A1.centre
  constraint coincident A2 A3.centre
  measures "d19" diameter of A2
  measures "d20" diameter of A3
extrude "Estrusione5" add sketch "Schizzo4" along normal blind 7 contours A2 A3 A4 A5 A6 A7 A8 A9 A10 A11 A12 A13 A14 A15 A16 A17 A18 A19 A20 A21 A22 A23 A24 A25 A26 A27 A28
sketch "Schizzo5" plane through (0, 0, 2) normal (0, 0, 1) x (-1, 0, 0)
  line L0 (-0.8, 1.833) -> (-0.8, 3.9192)
  arc A0 (0.8, 3.9192) -> (-0.8, 3.9192) centre (0, 0) ccw
  line L1 (0.8, 3.9192) -> (0.8, 1.833)
  arc A1 (0.8, -1.833) -> (0.8, 1.833) centre (0, 0) ccw
  line L2 (0.8, -1.833) -> (0.8, -3.9192)
  arc A2 (-0.8, -3.9192) -> (0.8, -3.9192) centre (0, 0) ccw
  line L3 (-0.8, -3.9192) -> (-0.8, -1.833)
  arc A3 (-0.8, 1.833) -> (-0.8, -1.833) centre (0, 0) ccw
  line L4 (-1, -5.9161) -> (-1, -15)
  line L5 (-1, -15) -> (1, -15)
  line L6 (1, -15) -> (1, -5.9161)
  arc A4 (1, -5.9161) -> (1, 5.9161) centre (0, 0) ccw
  line L7 (1, 5.9161) -> (1, 55)
  line L8 (1, 55) -> (-1, 55)
  line L9 (-1, 55) -> (-1, 5.9161)
  arc A5 (-1, 5.9161) -> (-1, -5.9161) centre (0, 0) ccw
extrude "Estrusione6" cut sketch "Schizzo5" against normal up to surface (2 mm away)
sketch "Schizzo6" plane through (0, 0, -7) normal (0, 0, -1) x (1, 0, 0)
  arc A0 (2.592, 3.6786) -> (2.5204, 3.728) centre (0, 0) ccw
  arc A1 (1.6363, 4.192) -> (2.5204, 3.728) centre (2.0913, 3.9846) ccw
  arc A2 (1.6363, 4.192) -> (1.555, 4.2228) centre (0, 0) ccw
  arc A3 (0.5856, 4.4617) -> (1.555, 4.2228) centre (1.0769, 4.3692) ccw
  arc A4 (0.5856, 4.4617) -> (0.4992, 4.4722) centre (0, 0) ccw
  arc A5 (-0.4992, 4.4722) -> (0.4992, 4.4722) centre (0, 4.5) ccw
  arc A6 (-0.4992, 4.4722) -> (-0.5856, 4.4617) centre (0, 0) ccw
  arc A7 (-1.555, 4.2228) -> (-0.5856, 4.4617) centre (-1.0769, 4.3692) ccw
  arc A8 (-1.555, 4.2228) -> (-1.6363, 4.192) centre (0, 0) ccw
  arc A9 (-2.5204, 3.728) -> (-1.6363, 4.192) centre (-2.0913, 3.9846) ccw
  arc A10 (-2.5204, 3.728) -> (-2.592, 3.6786) centre (0, 0) ccw
  arc A11 (-3.3393, 3.0165) -> (-2.592, 3.6786) centre (-2.9841, 3.3683) ccw
  arc A12 (-3.3393, 3.0165) -> (-3.397, 2.9514) centre (0, 0) ccw
  arc A13 (-3.9642, 2.1297) -> (-3.397, 2.9514) centre (-3.7034, 2.5563) ccw
  arc A14 (-3.9642, 2.1297) -> (-4.0046, 2.0527) centre (0, 0) ccw
  arc A15 (-4.3586, 1.1191) -> (-4.0046, 2.0527) centre (-4.2076, 1.5957) ccw
  arc A16 (-4.3586, 1.1191) -> (-4.3794, 1.0347) centre (0, 0) ccw
  arc A17 (-4.4998, 0.0435) -> (-4.3794, 1.0347) centre (-4.4672, 0.5424) ccw
  arc A18 (-4.4998, 0.0435) -> (-4.4998, -0.0435) centre (0, 0) ccw
  arc A19 (-4.3794, -1.0347) -> (-4.4998, -0.0435) centre (-4.4672, -0.5424) ccw
  arc A20 (-4.3794, -1.0347) -> (-4.3586, -1.1191) centre (0, 0) ccw
  arc A21 (-4.0046, -2.0527) -> (-4.3586, -1.1191) centre (-4.2076, -1.5957) ccw
  arc A22 (-4.0046, -2.0527) -> (-3.9642, -2.1297) centre (0, 0) ccw
  arc A23 (-3.397, -2.9514) -> (-3.9642, -2.1297) centre (-3.7034, -2.5563) ccw
  arc A24 (-3.397, -2.9514) -> (-3.3393, -3.0165) centre (0, 0) ccw
  arc A25 (-2.592, -3.6786) -> (-3.3393, -3.0165) centre (-2.9841, -3.3683) ccw
  arc A26 (-2.592, -3.6786) -> (-2.5204, -3.728) centre (0, 0) ccw
  arc A27 (-1.6363, -4.192) -> (-2.5204, -3.728) centre (-2.0913, -3.9846) ccw
  arc A28 (-1.6363, -4.192) -> (-1.555, -4.2228) centre (0, 0) ccw
  arc A29 (-0.5856, -4.4617) -> (-1.555, -4.2228) centre (-1.0769, -4.3692) ccw
  arc A30 (-0.5856, -4.4617) -> (-0.4992, -4.4722) centre (0, 0) ccw
  arc A31 (0.4992, -4.4722) -> (-0.4992, -4.4722) centre (0, -4.5) ccw
  arc A32 (0.4992, -4.4722) -> (0.5856, -4.4617) centre (0, 0) ccw
  arc A33 (1.555, -4.2228) -> (0.5856, -4.4617) centre (1.0769, -4.3692) ccw
  arc A34 (1.555, -4.2228) -> (1.6363, -4.192) centre (0, 0) ccw
  arc A35 (2.5204, -3.728) -> (1.6363, -4.192) centre (2.0913, -3.9846) ccw
  arc A36 (2.5204, -3.728) -> (2.592, -3.6786) centre (0, 0) ccw
  arc A37 (3.3393, -3.0165) -> (2.592, -3.6786) centre (2.9841, -3.3683) ccw
  arc A38 (3.3393, -3.0165) -> (3.397, -2.9514) centre (0, 0) ccw
  arc A39 (3.9642, -2.1297) -> (3.397, -2.9514) centre (3.7034, -2.5563) ccw
  arc A40 (3.9642, -2.1297) -> (4.0046, -2.0527) centre (0, 0) ccw
  arc A41 (4.3586, -1.1191) -> (4.0046, -2.0527) centre (4.2076, -1.5957) ccw
  arc A42 (4.3586, -1.1191) -> (4.3794, -1.0347) centre (0, 0) ccw
  arc A43 (4.4998, -0.0435) -> (4.3794, -1.0347) centre (4.4672, -0.5424) ccw
  arc A44 (4.4998, -0.0435) -> (4.4998, 0.0435) centre (0, 0) ccw
  arc A45 (4.3794, 1.0347) -> (4.4998, 0.0435) centre (4.4672, 0.5424) ccw
  arc A46 (4.3794, 1.0347) -> (4.3586, 1.1191) centre (0, 0) ccw
  arc A47 (4.0046, 2.0527) -> (4.3586, 1.1191) centre (4.2076, 1.5957) ccw
  arc A48 (4.0046, 2.0527) -> (3.9642, 2.1297) centre (0, 0) ccw
  arc A49 (3.397, 2.9514) -> (3.9642, 2.1297) centre (3.7034, 2.5563) ccw
  arc A50 (3.397, 2.9514) -> (3.3393, 3.0165) centre (0, 0) ccw
  arc A51 (2.592, 3.6786) -> (3.3393, 3.0165) centre (2.9841, 3.3683) ccw
  line L0 (-1.5, 8) -> (1.5, 8)
  line L1 (1.5, 8) -> (1.5, -40)
  line L2 (1.5, -40) -> (-1.5, -40)
  line L3 (-1.5, -40) -> (-1.5, 8)
  dimension "d27" = 8
  dimension "d28" = 40
  dimension "d29" = 3
  dimension "d30" = 1.5
  constraint horizontal L0
  constraint vertical L1
  constraint horizontal L2
  constraint vertical L3
  measures "d27" distance of A0.centre L0
  measures "d28" distance of A0.centre L2
  measures "d29" distance of L0.start L0.end
  measures "d30" distance of A0.centre L3
extrude "Estrusione7" [rolled back] along distance -9 taper angle 0
sketch "Schizzo7" plane through (0, 0, 0) normal (0, 0, 1) x (-1, 0, 0)
  line L0 (1.5, -1.3229) -> (1.5, -4.1028)
  arc A0 (1.555, -4.2228) -> (1.5, -4.1028) centre (1.0769, -4.3692) ccw
  arc A1 (1.555, -4.2228) -> (1.6363, -4.192) centre (0, 0) ccw
  arc A2 (2.5204, -3.728) -> (1.6363, -4.192) centre (2.0913, -3.9846) ccw
  arc A3 (2.5204, -3.728) -> (2.592, -3.6786) centre (0, 0) ccw
  arc A4 (3.3393, -3.0165) -> (2.592, -3.6786) centre (2.9841, -3.3683) ccw
  arc A5 (3.3393, -3.0165) -> (3.397, -2.9514) centre (0, 0) ccw
  arc A6 (3.9642, -2.1297) -> (3.397, -2.9514) centre (3.7034, -2.5563) ccw
  arc A7 (3.9642, -2.1297) -> (4.0046, -2.0527) centre (0, 0) ccw
  arc A8 (4.3586, -1.1191) -> (4.0046, -2.0527) centre (4.2076, -1.5957) ccw
  arc A9 (4.3586, -1.1191) -> (4.3794, -1.0347) centre (0, 0) ccw
  arc A10 (4.4998, -0.0435) -> (4.3794, -1.0347) centre (4.4672, -0.5424) ccw
  arc A11 (4.4998, -0.0435) -> (4.4998, 0.0435) centre (0, 0) ccw
  arc A12 (4.3794, 1.0347) -> (4.4998, 0.0435) centre (4.4672, 0.5424) ccw
  arc A13 (4.3794, 1.0347) -> (4.3586, 1.1191) centre (0, 0) ccw
  arc A14 (4.0046, 2.0527) -> (4.3586, 1.1191) centre (4.2076, 1.5957) ccw
  arc A15 (4.0046, 2.0527) -> (3.9642, 2.1297) centre (0, 0) ccw
  arc A16 (3.397, 2.9514) -> (3.9642, 2.1297) centre (3.7034, 2.5563) ccw
  arc A17 (3.397, 2.9514) -> (3.3393, 3.0165) centre (0, 0) ccw
  arc A18 (2.592, 3.6786) -> (3.3393, 3.0165) centre (2.9841, 3.3683) ccw
  arc A19 (2.592, 3.6786) -> (2.5204, 3.728) centre (0, 0) ccw
  arc A20 (1.6363, 4.192) -> (2.5204, 3.728) centre (2.0913, 3.9846) ccw
  arc A21 (1.6363, 4.192) -> (1.555, 4.2228) centre (0, 0) ccw
  arc A22 (1.5, 4.1028) -> (1.555, 4.2228) centre (1.0769, 4.3692) ccw
  line L1 (1.5, 4.1028) -> (1.5, 1.3229)
  arc A23 (1.5, -1.3229) -> (1.5, 1.3229) centre (0, 0) ccw
  circle A24 centre (0, 0) radius 5
  constraint coincident A1.centre A3.centre
extrude "Estrusione8" [rolled back] side1offset 0 taper angle 0

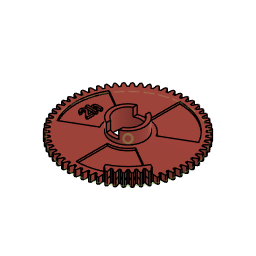
design "7 ore"
description: Spur Gear; Module: 0.930000; Num Teeth: 60; Pressure Angle: 20.000000; Backlash: 0.00 mm
Autodesk Fusion 360 part; units mm, degrees
sketch "Schizzo1" plane through (0, 0, 0) normal (0, 0, 1) x (1, 0, 0) in component "Spur Gear (60 teeth) (1)"
  circle A0 centre (0, 0) radius 26.7332
  circle A1 centre (0, 0) radius 4.1
extrude "Estrusione1" add sketch "Schizzo1" along normal blind 6 in component "Spur Gear (60 teeth) (1)"
sketch "Schizzo2" plane through (0, 0, 0) normal (0, 0, 1) x (1, 0, 0) in component "Spur Gear (60 teeth) (1)"
  spline S0 degree 5 poles (26.1953, -1.0768) (26.2029, -1.0768) (26.218, -1.0767) (26.2407, -1.0765) (26.271, -1.0757) (26.3089, -1.0742) (26.3468, -1.0722) (26.3847, -1.0696) (26.4226, -1.0664) (26.4605, -1.0628) (26.4984, -1.0587) (26.5363, -1.0542) (26.5742, -1.0494) (26.6121, -1.0443) (26.65, -1.0388) (26.6879, -1.0332) (26.7258, -1.0272) (26.7637, -1.0209) (26.8015, -1.0144) (26.8394, -1.0076) (26.8773, -1.0005) (26.9151, -0.9932) (26.953, -0.9856) (26.9908, -0.9778) (27.0286, -0.9697) (27.0664, -0.9615) (27.1042, -0.953) (27.142, -0.9443) (27.1798, -0.9354) (27.2176, -0.9262) (27.2553, -0.9169) (27.2931, -0.9073) (27.3308, -0.8976) (27.3686, -0.8876) (27.4063, -0.8775) (27.444, -0.8671) (27.4817, -0.8566) (27.5193, -0.8459) (27.557, -0.835) (27.5946, -0.8239) (27.6323, -0.8126) (27.6699, -0.8011) (27.7075, -0.7895) (27.7451, -0.7777) (27.7827, -0.7657) (27.8202, -0.7536) (27.8578, -0.7412) (27.8953, -0.7288) (27.9328, -0.7161) (27.9703, -0.7033) (28.0078, -0.6903) (28.0452, -0.6771) (28.0827, -0.6638) (28.1201, -0.6503) (28.1575, -0.6367) (28.1949, -0.6229) (28.2323, -0.609) (28.2697, -0.5949) (28.307, -0.5806) (28.3443, -0.5662) (28.3816, -0.5516) (28.4189, -0.5369) (28.4562, -0.522) (28.4934, -0.507) (28.5306, -0.4919) (28.5678, -0.4766) (28.605, -0.4611) (28.6422, -0.4455) (28.6793, -0.4298) (28.7164, -0.4139) (28.7535, -0.3978) (28.7832, -0.3849) (28.8055, -0.3751) (28.8203, -0.3686) (28.8277, -0.3653) knots 0 0 0 0 0 0 0.01428571 0.02857143 0.04285714 0.05714286 0.07142857 0.08571429 0.1 0.11428571 0.12857143 0.14285714 0.15714286 0.17142857 0.18571429 0.2 0.21428571 0.22857143 0.24285714 0.25714286 0.27142857 0.28571429 0.3 0.31428571 0.32857143 0.34285714 0.35714286 0.37142857 0.38571429 0.4 0.41428571 0.42857143 0.44285714 0.45714286 0.47142857 0.48571429 0.5 0.51428571 0.52857143 0.54285714 0.55714286 0.57142857 0.58571429 0.6 0.61428571 0.62857143 0.64285714 0.65714286 0.67142857 0.68571429 0.7 0.71428571 0.72857143 0.74285714 0.75714286 0.77142857 0.78571429 0.8 0.81428571 0.82857143 0.84285714 0.85714286 0.87142857 0.88571429 0.9 0.91428571 0.92857143 0.94285714 0.95714286 0.97142857 0.98571429 1 1 1 1 1 1
  spline S1 degree 5 poles (26.1953, 1.0768) (26.2029, 1.0768) (26.218, 1.0767) (26.2407, 1.0765) (26.271, 1.0757) (26.3089, 1.0742) (26.3468, 1.0722) (26.3847, 1.0696) (26.4226, 1.0664) (26.4605, 1.0628) (26.4984, 1.0587) (26.5363, 1.0542) (26.5742, 1.0494) (26.6121, 1.0443) (26.65, 1.0388) (26.6879, 1.0332) (26.7258, 1.0272) (26.7637, 1.0209) (26.8015, 1.0144) (26.8394, 1.0076) (26.8773, 1.0005) (26.9151, 0.9932) (26.953, 0.9856) (26.9908, 0.9778) (27.0286, 0.9697) (27.0664, 0.9615) (27.1042, 0.953) (27.142, 0.9443) (27.1798, 0.9354) (27.2176, 0.9262) (27.2553, 0.9169) (27.2931, 0.9073) (27.3308, 0.8976) (27.3686, 0.8876) (27.4063, 0.8775) (27.444, 0.8671) (27.4817, 0.8566) (27.5193, 0.8459) (27.557, 0.835) (27.5946, 0.8239) (27.6323, 0.8126) (27.6699, 0.8011) (27.7075, 0.7895) (27.7451, 0.7777) (27.7827, 0.7657) (27.8202, 0.7536) (27.8578, 0.7412) (27.8953, 0.7288) (27.9328, 0.7161) (27.9703, 0.7033) (28.0078, 0.6903) (28.0452, 0.6771) (28.0827, 0.6638) (28.1201, 0.6503) (28.1575, 0.6367) (28.1949, 0.6229) (28.2323, 0.609) (28.2697, 0.5949) (28.307, 0.5806) (28.3443, 0.5662) (28.3816, 0.5516) (28.4189, 0.5369) (28.4562, 0.522) (28.4934, 0.507) (28.5306, 0.4919) (28.5678, 0.4766) (28.605, 0.4611) (28.6422, 0.4455) (28.6793, 0.4298) (28.7164, 0.4139) (28.7535, 0.3978) (28.7832, 0.3849) (28.8055, 0.3751) (28.8203, 0.3686) (28.8277, 0.3653) knots 0 0 0 0 0 0 0.01428571 0.02857143 0.04285714 0.05714286 0.07142857 0.08571429 0.1 0.11428571 0.12857143 0.14285714 0.15714286 0.17142857 0.18571429 0.2 0.21428571 0.22857143 0.24285714 0.25714286 0.27142857 0.28571429 0.3 0.31428571 0.32857143 0.34285714 0.35714286 0.37142857 0.38571429 0.4 0.41428571 0.42857143 0.44285714 0.45714286 0.47142857 0.48571429 0.5 0.51428571 0.52857143 0.54285714 0.55714286 0.57142857 0.58571429 0.6 0.61428571 0.62857143 0.64285714 0.65714286 0.67142857 0.68571429 0.7 0.71428571 0.72857143 0.74285714 0.75714286 0.77142857 0.78571429 0.8 0.81428571 0.82857143 0.84285714 0.85714286 0.87142857 0.88571429 0.9 0.91428571 0.92857143 0.94285714 0.95714286 0.97142857 0.98571429 1 1 1 1 1 1
  arc A0 (28.8277, -0.3653) -> (28.8277, 0.3653) centre (0, 0) ccw
  line L0 (26.1953, 1.0768) -> (26.1953, -1.0768)
  point P0 (26.3824, -1.0696)
  point P1 (26.5699, -1.0499)
  point P2 (26.7578, -1.0218)
  point P3 (26.9458, -0.987)
  point P4 (27.134, -0.9461)
  point P5 (27.3223, -0.8997)
  point P6 (27.5106, -0.8483)
  point P7 (27.699, -0.7921)
  point P8 (27.8873, -0.7314)
  point P9 (28.0756, -0.6663)
  point P10 (28.2639, -0.597)
  point P11 (28.452, -0.5237)
  point P12 (28.6399, -0.4464)
  point P13 (26.3824, 1.0696)
  point P14 (26.5699, 1.0499)
  point P15 (26.7578, 1.0218)
  point P16 (26.9458, 0.987)
  point P17 (27.134, 0.9461)
  point P18 (27.3223, 0.8997)
  point P19 (27.5106, 0.8483)
  point P20 (27.699, 0.7921)
  point P21 (27.8873, 0.7314)
  point P22 (28.0756, 0.6663)
  point P23 (28.2639, 0.597)
  point P24 (28.452, 0.5237)
  point P25 (28.6399, 0.4464)
extrude "Estrusione2" add sketch "Schizzo2" along normal blind 6 in component "Spur Gear (60 teeth) (1)"
fillet "Raccordo1" radius 0.1 2 edges at (26.7134, 1.0291, 3) (26.7134, -1.0291, 3) in component "Spur Gear (60 teeth) (1)"
pattern_circular "Serie C1" count 60 over 360 about axis through (0, 0, 0) along (0, 0, 1) of "Estrusione2", "Raccordo1" in component "Spur Gear (60 teeth) (1)"
sketch "Schizzo3" plane through (0, 0, 0) normal (0, 0, 1) x (1, 0, 0) in component "Spur Gear (60 teeth) (1)"
  circle A0 centre (0, 0) radius 27.9 construction
extrude "Estrusione3" cut 1 faces at (19.1734, 0, 6) along direction (0, 0, -1) blind 3 in component "Spur Gear (60 teeth) (1)"